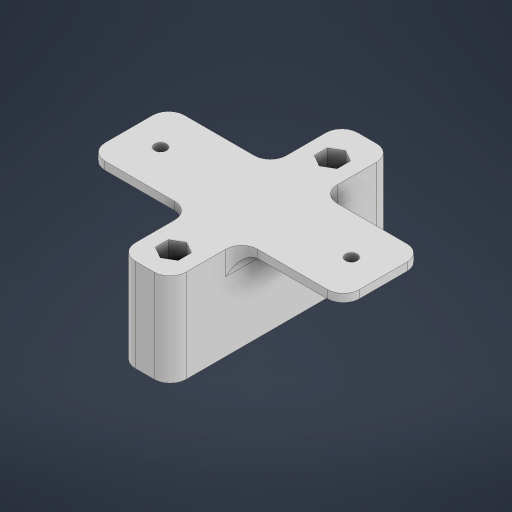
# Autodesk Inventor part: BRAIN_MOUNT
Saved by Autodesk Inventor 2024 (Build 280153000, 153)
## iProperties
Created: 2024-02-07
Part Number: BRAIN_MOUNT
Material: Generic
Document SubType Name: Modeling
Designer: eddy
Density: 1 g/cm^3
Appearance: Default
Author: eddy
Autodesk Inventor part; units mm, degrees
ref_plane "YZ Plane" through (0, 0, 0) normal (1, 0, 0) x (0, 1, 0)
ref_plane "XZ Plane" through (0, 0, 0) normal (0, 1, 0) x (-1, 0, 0)
ref_plane "XY Plane" through (0, 0, 0) normal (0, 0, 1) x (1, 0, 0)
sketch "Sketch1" plane through (0, 0, 0) normal (0, 1, 0) x (-1, 0, 0)
  line L0 (0, 0) -> (20.32, 0)
  line L1 (20.32, 0) -> (20.32, -88.9)
  line L2 (20.32, -88.9) -> (0, -88.9)
  line L3 (0, -88.9) -> (0, 0)
  line L4 (10.16, -88.9) -> (10.16, -74.93) construction
  circle A0 centre (10.16, -74.93) radius 2.3368
  circle A1 centre (10.16, -11.43) radius 2.3368
  dimension "d0" = 20.32
  dimension "d1" = 88.9
  dimension "d2" = 13.97
  dimension "d3" = 4.6736
  dimension "d4" = 63.5
  constraints: 10 end point, 2 centre point, 2 parallel, 1 coincident, 1 equal radius, 1 horizontal, 1 midpoint, 1 perpendicular, 1 point on line, 1 vertical
  measures "d0" distance of L1.end L2.end
  measures "d1" distance of L0.end L1.end
  measures "d2" distance of L4.start L4.end
  measures "d3" diameter of A0
  measures "d4" distance of A0.centre A1.centre
extrude "Extrusion1" add sketch "Sketch1" along normal blind 37.084
sketch "Sketch2" plane through (0, 37.084, 0) normal (0, 1, 0) x (1, 0, 0)
  line L0 (-60.96, 60.325) -> (40.64, 60.325)
  line L1 (40.64, 60.325) -> (40.64, 28.575)
  line L2 (40.64, 28.575) -> (-60.96, 28.575)
  line L3 (-60.96, 28.575) -> (-60.96, 60.325)
  line L4 (0, 88.9) -> (-20.32, 88.9) projected
  line L5 (-10.16, 60.325) -> (-10.16, 28.575)
  line L6 (-60.96, 44.45) -> (40.64, 44.45) construction
  circle A0 centre (-48.26, 44.45) radius 2.3368
  circle A1 centre (27.94, 44.45) radius 2.3368
  circle A2 centre (-10.16, 74.93) radius 2.3368 projected
  line L7 (-10.16, 88.9) -> (-10.16, 44.45)
  point P0 (0, 0)
  point P1 (-12.351, 76.2)
  point P2 (-15.843, 76.2)
  dimension "d8" = 31.75
  dimension "d9" = 101.6
  dimension "d11" = 4.6736
  dimension "d17" = 44.45
  dimension "d18" = 38.1
  dimension "d19" = 38.1
  constraints: 14 end point, 6 midpoint, 2 centre point, 2 parallel, 2 point on line, 1 collinear, 1 equal radius, 1 horizontal, 1 perpendicular
  measures "d8" distance of L0.end L1.end
  measures "d9" distance of L1.end L2.end
  measures "d11" diameter of A0
  measures "d17" distance of L7.start L7.end
  measures "d18" horizontal distance of A0.centre A2.centre
  measures "d19" horizontal distance of A1.centre A2.centre
extrude "Extrusion2" add sketch "Sketch2" against normal blind 3.175 contours L0 L5 L2 L3 | L0 L1 L2 L5
sketch "Sketch3" plane through (0, 37.084, 0) normal (0, 1, 0) x (1, 0, 0)
  circle A0 centre (-10.16, 11.43) radius 2.3368 projected
  circle A1 centre (-10.16, 11.43) radius 4.445
  circle A2 centre (-10.16, 74.93) radius 2.3368 projected
  circle A3 centre (-10.16, 74.93) radius 4.445
  point P0 (0, 0)
  dimension "d20" = 8.89
  constraints: 2 centre point, 2 coincident, 1 equal radius
  measures "d20" diameter of A1
extrude "Extrusion3" cut sketch "Sketch3" against normal blind 16.002 contours A0 | A1 | A2 | A3
fillet "Fillet1" radius 6.35 4 edges at (-20.32, 18.542, -88.9) (0, 18.542, -88.9) (-20.32, 18.542, 0) (0, 18.542, 0)
fillet "Fillet2" radius 6.35 8 edges at (-60.96, 35.4965, -60.325) (-60.96, 35.4965, -28.575) (-20.32, 35.4965, -28.575) (0, 35.4965, -28.575) (40.64, 35.4965, -28.575) (40.64, 35.4965, -60.325) (0, 35.4965, -60.325) (-20.32, 35.4965, -60.325)
fillet "Fillet3" radius 6.35 2 edges at (-20.32, 33.909, -44.45) (0, 33.909, -44.45)
sketch "Sketch4" plane through (0, 37.084, 0) normal (0, 1, 0) x (1, 0, 0)
  line L0 (-6.35, 88.9) -> (-13.97, 88.9) projected
  line L1 (-10.16, 88.9) -> (-10.16, 0)
  line L2 (-13.97, 0) -> (-6.35, 0) projected
  circle A0 centre (-10.16, 74.93) radius 2.3368 projected
  line L3 (-10.16, 80.1878) -> (-5.6066, 77.5589)
  line L4 (-5.6066, 77.5589) -> (-5.6066, 72.3011)
  line L5 (-5.6066, 72.3011) -> (-10.16, 69.6722)
  line L6 (-10.16, 69.6722) -> (-14.7134, 72.3011)
  line L7 (-14.7134, 72.3011) -> (-14.7134, 77.5589)
  line L8 (-14.7134, 77.5589) -> (-10.16, 80.1878)
  circle A1 centre (-10.16, 11.43) radius 2.3368 projected
  line L9 (-10.16, 16.6878) -> (-5.6066, 14.0589)
  line L10 (-5.6066, 14.0589) -> (-5.6066, 8.8011)
  line L11 (-5.6066, 8.8011) -> (-10.16, 6.1722)
  line L12 (-10.16, 6.1722) -> (-14.7134, 8.8011)
  line L13 (-14.7134, 8.8011) -> (-14.7134, 14.0589)
  line L14 (-14.7134, 14.0589) -> (-10.16, 16.6878)
  point P0 (0, 0)
  dimension "d26" = 5.2578
  dimension "d27" = 5.2578
  constraints: 26 end point, 2 coincident, 2 midpoint, 2 point on line, 26 other
  measures "d26" distance of L3.end L4.end
  measures "d27" distance of L9.end L10.end
extrude "Extrusion4" cut sketch "Sketch4" against normal up to surface (16.002 mm away) contours L9 L10 L11 L1 A1 | L1 A1 L12 L13 L14 | L6 L7 L8 L1 A0 | L1 A0 L3 L4 L5
body "Solid1"
